Autodesk Fusion 360 part; units mm, degrees
(part 2 of 18)
  line L906 (81.5823, -43.3625) -> (81.9887, -43.0894)
  line L907 (120.3611, -22.6739) -> (127.5638, -15.4712)
  line L908 (99.6621, -41.0408) -> (99.2557, -41.3139)
  line L909 (101.3111, -22.6739) -> (109.1488, -14.8362)
  line L910 (99.2557, -41.3139) -> (98.9843, -41.7214)
  line L911 (62.5323, -60.1036) -> (62.5323, -43.3625)
  line L912 (137.0841, -23.6313) -> (137.3555, -24.0392)
  line L913 (44.2552, -61.2644) -> (44.16, -60.7842)
  line L914 (137.3569, -22.2627) -> (137.0849, -22.6702)
  line L915 (137.3558, -60.3767) -> (137.0844, -60.7842)
  line L916 (81.9887, -43.0894) -> (82.26, -42.6819)
  line L917 (81.9887, -41.3139) -> (81.5823, -41.0408)
  line L918 (117.9391, -23.1507) -> (118.0341, -23.6313)
  line L919 (118.0349, -22.6702) -> (117.9391, -23.1507)
  line L920 (63.3053, -23.1536) -> (63.211, -22.6739)
  line L921 (138.7251, -21.9878) -> (138.2443, -21.8935)
  line L922 (61.562, -43.3625) -> (61.562, -60.1036)
  line L923 (60.8842, -42.6819) -> (61.1556, -43.0894)
  line L924 (42.9971, -81.5853) -> (43.478, -81.4897)
  line L925 (137.0844, -42.6819) -> (137.3558, -43.0894)
  line L926 (61.1556, -60.3767) -> (60.8842, -60.7842)
  line L927 (117.9391, -61.2644) -> (118.0344, -61.7447)
  line L928 (118.0344, -61.7447) -> (118.3057, -62.1522)
  line L929 (118.3052, -79.4399) -> (118.0338, -79.8483)
  line L930 (43.4822, -60.1036) -> (43.4822, -43.3625)
  line L931 (71.8355, -12.6772) -> (62.5249, -21.9878)
  line L932 (98.9843, -61.7447) -> (99.2557, -62.1522)
  line L933 (98.9843, -60.7842) -> (98.8891, -61.2644)
  line L934 (99.2557, -60.3767) -> (98.9843, -60.7842)
  line L935 (99.6621, -43.3625) -> (99.6621, -60.1036)
  line L936 (99.6621, -60.1036) -> (99.2557, -60.3767)
  line L937 (118.7121, -62.4253) -> (118.7121, -79.1663)
  line L938 (99.2555, -24.0392) -> (99.6621, -24.3125)
  line L939 (118.7121, -79.1663) -> (118.3052, -79.4399)
  line L940 (62.9386, -62.1522) -> (63.21, -61.7447)
  line L941 (119.6824, -62.4253) -> (120.0888, -62.1522)
  line L942 (43.8886, -60.3767) -> (43.4822, -60.1036)
  line L943 (42.5119, -79.1663) -> (42.105, -79.4399)
  line L944 (136.9891, -42.2017) -> (137.0844, -42.6819)
  line L945 (98.8891, -61.2644) -> (98.9843, -61.7447)
  line L946 (119.6824, -41.0408) -> (119.6824, -24.3125)
  line L947 (119.6824, -79.1663) -> (119.6824, -62.4253)
  line L948 (120.0888, -62.1522) -> (120.3601, -61.7447)
  line L949 (62.5323, -24.3125) -> (62.9382, -24.0399)
  line L950 (138.2473, -81.5853) -> (138.7282, -81.4897)
  line L951 (63.21, -42.6819) -> (63.3053, -42.2017)
  line L952 (23.0555, -62.1522) -> (23.4619, -62.4253)
  line L953 (23.0555, -60.3767) -> (22.7842, -60.7842)
  line L954 (42.5138, -21.99) -> (42.1067, -22.2627)
  line L955 (24.4322, -41.0408) -> (24.4322, -24.3125)
  line L956 (178.6173, -0.7849) -> (176.3475, -0.7849)
  line L957 (25.2052, -23.1536) -> (25.1109, -22.6739)
  line L958 (23.4661, -81.4897) -> (23.947, -81.5853)
  line L959 (213.072, -5.8134) -> (212.8706, -6.0548)
  line L960 (24.8386, -41.3139) -> (24.4322, -41.0408)
  line L961 (25.2052, -42.2017) -> (25.1099, -41.7214)
  line L962 (41.8342, -60.7842) -> (41.7389, -61.2644)
  line L963 (200.216, -3.6301) -> (200.443, -3.4264)
  line L964 (194.0618, -4.9249) -> (193.7985, -4.9771)
  line L965 (42.1056, -43.0894) -> (42.5119, -43.3625)
  line L966 (4.897, -81.5853) -> (5.378, -81.4897)
  line L967 (176.8325, -43.3625) -> (177.2389, -43.0894)
  line L968 (195.4081, -3.5504) -> (195.6982, -3.4341)
  line L969 (16.129, -12.8042) -> (16.3147, -12.7672)
  line L970 (4.0055, -43.0894) -> (4.4119, -43.3625)
  line L971 (208.5286, -4.7436) -> (208.3683, -4.4841)
  line L972 (172.9629, -1.8839) -> (172.9618, -2.1747)
  line L973 (3.7341, -42.6819) -> (4.0055, -43.0894)
  line L974 (-0.1723, -11.2229) -> (0.0069, -11.7151)
  line L975 (3.7341, -41.7214) -> (3.6389, -42.2017)
  line L976 (215.4944, -11.621) -> (215.6027, -11.9249)
  line L977 (193.4348, -5.3569) -> (190.7733, -5.3569)
  line L978 (200.4816, 0.4328) -> (194.6816, -5.3671)
  line L979 (5.3763, -21.9884) -> (4.8954, -21.8935)
  line L980 (194.9024, -6.8777) -> (201.168, -0.6121)
  line L981 (4.4119, -41.0408) -> (4.0055, -41.3139)
  line L982 (181.9207, 0.92) -> (181.5565, 1.0954)
  line L983 (23.4619, -60.1036) -> (23.0555, -60.3767)
  line L984 (24.428, -81.4897) -> (24.8359, -81.2176)
  line L985 (22.7842, -60.7842) -> (22.6889, -61.2644)
  line L986 (214.101, -6.1558) -> (213.9416, -5.8848)
  line L987 (24.4322, -24.3125) -> (24.8381, -24.0399)
  line L988 (41.8347, -22.6702) -> (41.7389, -23.1507)
  line L989 (216.7062, -11.9249) -> (216.8145, -11.621)
  line L990 (25.1099, -42.6819) -> (25.2052, -42.2017)
  line L991 (203.0295, -6.6507) -> (203.0804, -6.516)
  line L992 (24.4322, -43.3625) -> (24.8386, -43.0894)
  line L993 (25.2052, -80.3294) -> (25.1105, -79.8483)
  line L994 (41.7389, -61.2644) -> (41.8342, -61.7447)
  line L995 (174.114, -1.6018) -> (173.8815, -1.4273)
  line L996 (198.1398, 0.2231) -> (197.8664, 0.2821)
  line L997 (15.9233, -2.4518) -> (15.9041, -2.4514)
  line L998 (173.0884, -1.6216) -> (172.9629, -1.8839)
  line L999 (9.18, -6.8394) -> (8.7726, -7.1123)
  line L1000 (175.2949, -0.9886) -> (175.2326, -1.2915)
  line L1001 (4.0055, -62.1522) -> (4.4119, -62.4253)
  line L1002 (4.0082, -81.2176) -> (4.4161, -81.4897)
  line L1003 (18.072, -9.69) -> (15.9281, -11.8339)
  line L1004 (15.9041, -2.4514) -> (10.8302, -2.4514)
  line L1005 (167.1355, -6.8777) -> (166.9498, -6.9146)
  line L1006 (5.7885, -60.3767) -> (5.3822, -60.1036)
  line L1007 (172.2242, -5.218) -> (172.2313, -5.2888)
  line L1008 (196.8625, -6.7799) -> (196.7084, -6.805)
  line L1009 (8.4049, -8.0011) -> (8.5005, -8.4821)
  line L1010 (195.9027, -3.1978) -> (195.9764, -2.8941)
  line L1011 (4.4119, -62.4253) -> (4.4119, -79.1663)
  line L1012 (3.5508, -9.552) -> (3.0129, -9.4529)
  line L1013 (195.0968, -2.2673) -> (194.8337, -2.436)
  line L1014 (3.7341, -60.7842) -> (3.6389, -61.2644)
  line L1015 (22.7842, -42.6819) -> (23.0555, -43.0894)
  line L1016 (23.0555, -43.0894) -> (23.4619, -43.3625)
  line L1017 (23.4619, -43.3625) -> (23.4619, -60.1036)
  line L1018 (190.7733, -5.3569) -> (190.8695, -5.1322)
  line L1019 (195.0969, -3.521) -> (195.4081, -3.5504)
  line L1020 (41.7389, -42.2017) -> (41.8342, -42.6819)
  line L1021 (207.9228, -5.6157) -> (208.217, -5.5352)
  line L1022 (0.0069, -10.2069) -> (-0.1723, -10.6991)
  line L1023 (180.7794, -1.2929) -> (179.3263, -1.2929)
  line L1024 (190.9024, -3.7901) -> (190.8739, -3.5643)
  line L1025 (15.9424, -2.453) -> (15.9233, -2.4518)
  line L1026 (190.9024, -4.8901) -> (190.9024, -3.7901)
  line L1027 (22.7842, -41.7214) -> (22.6889, -42.2017)
  line L1028 (23.0555, -41.3139) -> (22.7842, -41.7214)
  line L1029 (22.6889, -42.2017) -> (22.7842, -42.6819)
  line L1030 (174.2496, -1.8591) -> (174.114, -1.6018)
  line L1031 (25.1099, -41.7214) -> (24.8386, -41.3139)
  line L1032 (43.4749, -21.9878) -> (42.9941, -21.8935)
  line L1033 (24.4322, -60.1036) -> (24.4322, -43.3625)
  line L1034 (42.1056, -60.3767) -> (41.8342, -60.7842)
  line L1035 (25.1099, -60.7842) -> (24.8386, -60.3767)
  line L1036 (175.2326, -1.2915) -> (175.3144, -1.5898)
  line L1037 (41.8342, -42.6819) -> (42.1056, -43.0894)
  line L1038 (3.6389, -61.2644) -> (3.7341, -61.7447)
  line L1039 (200.6801, 0.5655) -> (200.4816, 0.4328)
  line L1040 (165.1589, -8.4494) -> (165.3162, -8.3442)
  line L1041 (214.3747, -7.2577) -> (214.245, -6.9577)
  line L1042 (3.6389, -80.3294) -> (3.7353, -80.8102)
  line L1043 (5.7891, -79.4399) -> (5.3822, -79.1663)
  line L1044 (15.9425, -3.3693) -> (172.2299, -3.3545)
  line L1045 (198.1837, -6.3551) -> (198.1618, -6.6507)
  line L1046 (172.2242, -3.418) -> (172.2242, -5.218)
  line L1047 (182.2626, -0.59) -> (182.2626, 0.21)
  line L1048 (166.7893, -5.499) -> (164.7723, -7.516)
  line L1049 (5.3822, -43.3625) -> (5.7885, -43.0894)
  line L1050 (6.0599, -60.7842) -> (5.7885, -60.3767)
  line L1051 (16.3147, -12.7672) -> (16.4721, -12.6621)
  line L1052 (198.3525, -0.832) -> (198.7028, -0.925)
  line L1053 (200.1078, -2.4188) -> (199.8039, -2.3916)
  line L1054 (10.1698, -4.0727) -> (10.5742, -3.7888)
  line L1055 (175.7693, -0.6189) -> (175.4878, -0.7469)
  line L1056 (8.5005, -7.5202) -> (8.4049, -8.0011)
  line L1057 (201.688, -1.6181) -> (201.9182, -1.8376)
  line L1058 (23.4619, -24.3125) -> (23.4619, -41.0408)
  line L1059 (5.3822, -41.0408) -> (5.3822, -24.3125)
  line L1060 (22.6889, -80.3294) -> (22.7853, -80.8102)
  line L1061 (23.4619, -41.0408) -> (23.0555, -41.3139)
  line L1062 (197.8664, 0.2821) -> (197.593, 0.2231)
  line L1063 (195.6982, -3.4341) -> (195.9027, -3.1978)
  line L1064 (24.8386, -43.0894) -> (25.1099, -42.6819)
  line L1065 (25.2052, -61.2644) -> (25.1099, -60.7842)
  line L1066 (193.1903, -1.5521) -> (196.8003, -1.5521)
  line L1067 (5.7858, -81.2176) -> (6.0587, -80.8102)
  line L1068 (216.7666, -1.143) -> (216.72, -0.9087)
  line L1069 (179.3263, -1.2929) -> (178.9604, -0.927)
  line L1070 (197.3185, -1.8559) -> (197.6227, -1.8022)
  line L1071 (208.217, -5.5352) -> (208.444, -5.3314)
  line L1072 (216.72, -0.9087) -> (216.5873, -0.7102)
  line L1073 (3.7353, -80.8102) -> (4.0082, -81.2176)
  line L1074 (4.2428, -11.8339) -> (4.4732, -11.3379)
  line L1075 (203.1744, -2.8751) -> (203.3317, -2.9802)
  line L1076 (6.0599, -42.6819) -> (6.1552, -42.2017)
  line L1077 (42.5119, -43.3625) -> (42.5119, -60.1036)
  line L1078 (4.005, -79.4399) -> (3.7336, -79.8483)
  line L1079 (204.1263, -4.4896) -> (203.8403, -4.439)
  line L1080 (18.616, -10.5182) -> (19.9512, -10.5182)
  line L1081 (10.8302, -2.4514) -> (10.5593, -2.0381)
  line L1082 (198.3322, -6.0986) -> (198.1837, -6.3551)
  line L1083 (22.6889, -23.1507) -> (22.7839, -23.6313)
  line L1084 (53.5475, -11.9152) -> (43.4749, -21.9878)
  line L1085 (22.7839, -23.6313) -> (23.0553, -24.0392)
  line L1086 (8.7858, -3.823) -> (9.2008, -4.0913)
  line L1087 (4.0051, -24.039) -> (4.4119, -24.3125)
  line L1088 (24.8386, -62.1522) -> (25.1099, -61.7447)
  line L1089 (10.1419, -9.1646) -> (10.5503, -8.8932)
  line L1090 (24.8386, -60.3767) -> (24.4322, -60.1036)
  line L1091 (23.947, -81.5853) -> (24.428, -81.4897)
  line L1092 (41.8342, -41.7214) -> (41.7389, -42.2017)
  line L1093 (24.4322, -62.4253) -> (24.8386, -62.1522)
  line L1094 (198.0055, -1.3392) -> (198.001, -1.0303)
  line L1095 (5.3822, -60.1036) -> (5.3822, -43.3625)
  line L1096 (6.1552, -61.2644) -> (6.0599, -60.7842)
  line L1097 (5.3822, -79.1663) -> (5.3822, -62.4253)
  line L1098 (180.7882, 0.92) -> (180.5363, 0.6041)
  line L1099 (197.0968, -6.5566) -> (196.8881, -6.7799)
  line L1100 (176.0783, -0.6326) -> (175.7693, -0.6189)
  line L1101 (196.8003, -1.5521) -> (197.023, -1.7661)
  line L1102 (6.0605, -79.8483) -> (5.7891, -79.4399)
  line L1103 (198.3692, -3.9434) -> (198.3322, -4.129)
  line L1104 (200.3673, -2.5791) -> (200.1078, -2.4188)
  line L1105 (3.0129, -9.4529) -> (1.3129, -9.4529)
  line L1106 (16.4721, -12.6621) -> (18.616, -10.5182)
  line L1107 (23.4619, -62.4253) -> (23.4619, -79.1663)
  line L1108 (214.7579, -0.6121) -> (215.5423, -1.3966)
  line L1109 (205.667, -3.1846) -> (205.9467, -3.063)
  line L1110 (42.5119, -60.1036) -> (42.1056, -60.3767)
  line L1111 (4.4119, -43.3625) -> (4.4119, -60.1036)
  line L1112 (189.4281, 0.92) -> (189.1761, 0.6041)
  line L1113 (6.0587, -80.8102) -> (6.1552, -80.3294)
  line L1114 (197.3834, -6.4506) -> (197.0968, -6.5566)
  line L1115 (214.245, -6.9577) -> (213.9877, -6.7562)
  line L1116 (25.1109, -22.6739) -> (35.8696, -11.9152)
  line L1117 (22.7836, -79.8483) -> (22.6889, -80.3294)
  line L1118 (35.8696, -11.9152) -> (53.5475, -11.9152)
  line L1119 (24.8391, -79.4399) -> (24.4322, -79.1663)
  line L1120 (42.9941, -21.8935) -> (42.5138, -21.99)
  line L1121 (10.5742, -3.7888) -> (10.8381, -3.3709)
  line L1122 (25.1099, -61.7447) -> (25.2052, -61.2644)
  line L1123 (25.1105, -79.8483) -> (24.8391, -79.4399)
  line L1124 (42.5119, -41.0408) -> (42.1056, -41.3139)
  line L1125 (5.7885, -43.0894) -> (6.0599, -42.6819)
  line L1126 (200.5548, -3.1425) -> (200.5276, -2.8386)
  line L1127 (195.9764, -2.8941) -> (195.9027, -2.5903)
  line L1128 (199.2151, 0.1448) -> (198.923, 0.3594)
  line L1129 (6.1552, -80.3294) -> (6.0605, -79.8483)
  line L1130 (5.7885, -62.1522) -> (6.0599, -61.7447)
  line L1131 (206.1424, -2.2351) -> (205.9467, -2.0011)
  line L1132 (5.7844, -22.2598) -> (5.3763, -21.9884)
  line L1133 (8.405, -2.9318) -> (8.5061, -3.4155)
  line L1134 (10.8239, -7.516) -> (10.5503, -7.1091)
  line L1135 (201.828, -0.7484) -> (201.637, -1.0027)
  line L1136 (24.8381, -24.0399) -> (25.1094, -23.6331)
  line L1137 (197.023, -1.7661) -> (197.3185, -1.8559)
  line L1138 (194.8337, -2.436) -> (192.3062, -2.4363)
  line L1139 (42.5119, -24.3125) -> (42.5119, -41.0408)
  line L1140 (194.5428, -5.1373) -> (194.3243, -4.9814)
  line L1141 (3.7336, -79.8483) -> (3.6389, -80.3294)
  line L1142 (0.0069, -11.7151) -> (0.3435, -12.1163)
  line L1143 (18.415, -9.5479) -> (18.2294, -9.5848)
  line L1144 (203.7184, -2.0469) -> (202.9101, -1.2386)
  line L1145 (22.7847, -22.6702) -> (22.6889, -23.1507)
  line L1146 (205.9467, -2.0011) -> (205.667, -1.8794)
  line L1147 (23.4619, -79.1663) -> (23.055, -79.4399)
  line L1148 (4.4119, -60.1036) -> (4.0055, -60.3767)
  line L1149 (191.6477, 0.1862) -> (191.4903, 0.081)
  line L1150 (180.4463, 0.21) -> (180.4463, -0.59)
  line L1151 (6.0599, -41.7214) -> (5.7885, -41.3139)
  line L1152 (196.7084, -6.805) -> (196.5703, -6.8777)
  line L1153 (189.2636, -6.5975) -> (189.3011, -6.8777)
  line L1154 (23.4637, -21.99) -> (23.0567, -22.2627)
  line L1155 (23.9441, -21.8935) -> (23.4637, -21.99)
  line L1156 (23.055, -79.4399) -> (22.7836, -79.8483)
  line L1157 (23.0553, -24.0392) -> (23.4619, -24.3125)
  line L1158 (215.4443, 0.4328) -> (215.2457, 0.5655)
  line L1159 (42.1056, -41.3139) -> (41.8342, -41.7214)
  line L1160 (198.5618, 0.3884) -> (198.2393, 0.2231)
  line L1161 (202.1153, -0.6121) -> (201.828, -0.7484)
  line L1162 (8.5061, -3.4155) -> (8.7858, -3.823)
  line L1163 (216.4673, -12.1417) -> (216.7062, -11.9249)
  line L1164 (23.0582, -81.2176) -> (23.4661, -81.4897)
  line L1165 (23.0567, -22.2627) -> (22.7847, -22.6702)
  line L1166 (34.9975, -11.4151) -> (24.4248, -21.9878)
  line L1167 (22.7853, -80.8102) -> (23.0582, -81.2176)
  line L1168 (9.6871, -4.179) -> (10.1698, -4.0727)
  line L1169 (41.834, -23.6313) -> (42.1053, -24.0392)
  line L1170 (199.3507, -0.1912) -> (199.2151, 0.1448)
  line L1171 (175.4878, -0.7469) -> (175.2949, -0.9886)
  line L1172 (196.8881, -6.7799) -> (196.8625, -6.7799)
  line L1173 (1.3129, -9.4529) -> (0.7971, -9.5438)
  line L1174 (199.3163, -2.7304) -> (199.2357, -3.0246)
  line L1175 (24.4248, -21.9878) -> (23.9441, -21.8935)
  line L1176 (23.7467, -11.4151) -> (34.9975, -11.4151)
  line L1177 (23.5871, -11.4421) -> (23.6681, -11.4353)
  line L1178 (182.1727, 0.6041) -> (181.9207, 0.92)
  line L1179 (197.9434, -6.6507) -> (197.6871, -6.4844)
  line L1180 (41.7389, -23.1507) -> (41.834, -23.6313)
  line L1181 (6.0599, -61.7447) -> (6.1552, -61.2644)
  line L1182 (215.2457, 0.5655) -> (215.0114, 0.6121)
  line L1183 (198.4743, -3.786) -> (198.3692, -3.9434)
  line L1184 (3.1779, -12.6621) -> (3.3353, -12.7672)
  line L1185 (23.6681, -11.4353) -> (23.7467, -11.4151)
  line L1186 (20.3591, -11.4421) -> (23.5871, -11.4421)
  line L1187 (8.1491, -23.5999) -> (8.3065, -23.4947)
  line L1188 (25.1094, -23.6331) -> (25.2052, -23.1536)
  line L1189 (203.7228, -4.386) -> (203.5951, -4.3679)
  line L1190 (208.1088, -4.3238) -> (207.8049, -4.2966)
  line L1191 (193.5774, -5.1294) -> (193.4348, -5.3569)
  line L1192 (9.18, -9.1629) -> (9.6608, -9.2593)
  line L1193 (9.6608, -6.743) -> (9.18, -6.8394)
  line L1194 (7.7625, -22.6665) -> (6.0579, -22.6665)
  line L1195 (199.9607, -4.0327) -> (199.7531, -4.2406)
  line L1196 (10.5593, -2.0381) -> (10.1501, -1.7611)
  line L1197 (166.9467, -5.3938) -> (166.7893, -5.499)
  line L1198 (7.9634, -23.6368) -> (8.1491, -23.5999)
  line L1199 (8.3065, -23.4947) -> (20.3591, -11.4421)
  line L1200 (22.7842, -61.7447) -> (23.0555, -62.1522)
  line L1201 (207.1669, -6.1706) -> (207.3526, -6.1337)
  line L1202 (200.7795, -4.1206) -> (200.5297, -3.9662)
  line L1203 (42.1053, -24.0392) -> (42.5119, -24.3125)
  line L1204 (198.923, 0.3594) -> (198.5618, 0.3884)
  line L1205 (6.1552, -42.2017) -> (6.0599, -41.7214)
  line L1206 (4.4119, -79.1663) -> (4.005, -79.4399)
  line L1207 (174.3183, -1.9279) -> (174.2496, -1.8591)
  line L1208 (207.2367, -4.9296) -> (206.966, -5.2003)
  line L1209 (3.7337, -23.6309) -> (4.0051, -24.039)
  line L1210 (5.7867, -24.0413) -> (6.0579, -23.6368)
  line L1211 (5.3822, -24.3125) -> (5.7867, -24.0413)
  line L1212 (22.6889, -61.2644) -> (22.7842, -61.7447)
  line L1213 (4.0179, -9.8365) -> (3.5508, -9.552)
  line L1214 (25.1088, -80.8102) -> (25.2052, -80.3294)
  line L1215 (4.0055, -60.3767) -> (3.7341, -60.7842)
  line L1216 (24.4322, -79.1663) -> (24.4322, -62.4253)
  line L1217 (24.8359, -81.2176) -> (25.1088, -80.8102)
  line L1218 (42.1067, -22.2627) -> (41.8347, -22.6702)
  line L1219 (207.5211, -4.4084) -> (207.3173, -4.6354)
  line L1220 (203.5951, -4.3679) -> (200.9382, -4.3679)
  line L1221 (189.0861, -0.59) -> (189.1736, -0.9789)
  line L1222 (5.3822, -62.4253) -> (5.7885, -62.1522)
  line L1223 (203.0804, -6.516) -> (203.1011, -6.3734)
  line L1224 (191.8334, 0.2231) -> (191.6477, 0.1862)
  line L1225 (212.803, -6.3619) -> (212.5142, -6.6507)
  line L1226 (213.8751, -8.0076) -> (214.1642, -7.8552)
  line L1227 (4.4732, -11.3379) -> (4.5116, -10.7923)
  line L1228 (3.7341, -61.7447) -> (4.0055, -62.1522)
  line L1229 (173.0851, -2.4381) -> (15.9424, -2.453)
  line L1230 (5.378, -81.4897) -> (5.7858, -81.2176)
  line L1231 (192.3062, -2.4363) -> (193.1903, -1.5521)
  line L1232 (19.879, -10.5602) -> (19.8151, -10.6139)
  line L1233 (206.1424, -2.8289) -> (206.2125, -2.532)
  line L1234 (0.3435, -9.8057) -> (0.0069, -10.2069)
  line L1235 (6.0579, -23.6368) -> (7.9634, -23.6368)
  line L1236 (4.4161, -81.4897) -> (4.897, -81.5853)
  line L1237 (203.5174, -3.0171) -> (205.0973, -3.0171)
  line L1238 (5.7885, -41.3139) -> (5.3822, -41.0408)
  line L1239 (189.4193, -1.2929) -> (181.9295, -1.2929)
  line L1240 (213.362, -5.6919) -> (213.072, -5.8134)
  line L1241 (4.3529, -10.2689) -> (4.0179, -9.8365)
  line L1242 (1.8785, -81.4188) -> (1.397, -81.323)
  line L1243 (0.5074, -81.6915) -> (0.2346, -82.0997)
  line L1244 (0.9155, -83.7435) -> (1.397, -83.8393)
  line L1245 (2.5594, -82.0997) -> (2.2866, -81.6915)
  line L1246 (1.397, -81.323) -> (0.9155, -81.4188)
  line L1247 (2.2866, -83.4708) -> (2.5594, -83.0626)
  line L1248 (1.397, -83.8393) -> (1.8785, -83.7435)
  line L1249 (2.6551, -82.5812) -> (2.5594, -82.0997)
  line L1250 (0.1389, -82.5812) -> (0.2346, -83.0626)
  line L1251 (0.2346, -82.0997) -> (0.1389, -82.5812)
  line L1252 (0.2346, -83.0626) -> (0.5074, -83.4708)
  line L1253 (1.8785, -83.7435) -> (2.2866, -83.4708)
  line L1254 (2.2866, -81.6915) -> (1.8785, -81.4188)
  line L1255 (2.5594, -83.0626) -> (2.6551, -82.5812)
  line L1256 (0.5074, -83.4708) -> (0.9155, -83.7435)
  line L1257 (0.9155, -81.4188) -> (0.5074, -81.6915)
  line L1258 (1.8785, -64.6808) -> (2.2866, -64.4081)
  line L1259 (0.5074, -64.4081) -> (0.9155, -64.6808)
  line L1260 (2.2866, -62.6288) -> (1.8785, -62.3561)
  line L1261 (0.5074, -62.6288) -> (0.2346, -63.037)
  line L1262 (2.6551, -63.5184) -> (2.5594, -63.037)
  line L1263 (2.5594, -63.9999) -> (2.6551, -63.5184)
  line L1264 (0.2346, -63.037) -> (0.1389, -63.5184)
  line L1265 (0.2346, -63.9999) -> (0.5074, -64.4081)
  line L1266 (0.9155, -64.6808) -> (1.397, -64.7766)
  line L1267 (2.5594, -63.037) -> (2.2866, -62.6288)
  line L1268 (0.1389, -63.5184) -> (0.2346, -63.9999)
  line L1269 (0.9155, -62.3561) -> (0.5074, -62.6288)
  line L1270 (1.8785, -62.3561) -> (1.397, -62.2603)
  line L1271 (1.397, -64.7766) -> (1.8785, -64.6808)
  line L1272 (2.2866, -64.4081) -> (2.5594, -63.9999)
  line L1273 (1.397, -62.2603) -> (0.9155, -62.3561)
  line L1274 (0.5074, -26.2953) -> (0.9155, -26.568)
  line L1275 (0.9155, -26.568) -> (1.397, -26.6638)
  line L1276 (2.2866, -24.516) -> (1.8785, -24.2433)
  line L1277 (2.5594, -24.9242) -> (2.2866, -24.516)
  line L1278 (0.2346, -24.9242) -> (0.1389, -25.4057)
  line L1279 (1.397, -24.1475) -> (0.9155, -24.2433)
  line L1280 (0.9155, -24.2433) -> (0.5074, -24.516)
  line L1281 (1.397, -26.6638) -> (1.8785, -26.568)
  line L1282 (2.2866, -26.2953) -> (2.5594, -25.8871)
  line L1283 (2.6551, -25.4057) -> (2.5594, -24.9242)
  line L1284 (1.8785, -26.568) -> (2.2866, -26.2953)
  line L1285 (0.5074, -24.516) -> (0.2346, -24.9242)
  line L1286 (1.8785, -24.2433) -> (1.397, -24.1475)
  line L1287 (2.5594, -25.8871) -> (2.6551, -25.4057)
  line L1288 (0.2346, -25.8871) -> (0.5074, -26.2953)
  line L1289 (0.1389, -25.4057) -> (0.2346, -25.8871)
  line L1290 (2.5594, -44.9372) -> (2.6551, -44.4557)
  line L1291 (0.5074, -43.566) -> (0.2346, -43.9742)
  line L1292 (2.2866, -43.566) -> (1.8785, -43.2933)
  line L1293 (1.8785, -45.6181) -> (2.2866, -45.3453)
  line L1294 (0.2346, -43.9742) -> (0.1389, -44.4557)
  line L1295 (0.9155, -45.6181) -> (1.397, -45.7138)
  line L1296 (2.2866, -45.3453) -> (2.5594, -44.9372)
  line L1297 (1.397, -43.1975) -> (0.9155, -43.2933)
  line L1298 (0.5074, -45.3453) -> (0.9155, -45.6181)
  line L1299 (0.2346, -44.9372) -> (0.5074, -45.3453)
  line L1300 (1.397, -45.7138) -> (1.8785, -45.6181)
  line L1301 (0.1389, -44.4557) -> (0.2346, -44.9372)
  line L1302 (2.6551, -44.4557) -> (2.5594, -43.9742)
  line L1303 (2.5594, -43.9742) -> (2.2866, -43.566)
  line L1304 (1.8785, -43.2933) -> (1.397, -43.1975)
  line L1305 (0.9155, -43.2933) -> (0.5074, -43.566)
  line L1306 (9.1816, -4.2988) -> (8.7734, -4.5715)
  line L1307 (10.9212, -5.4611) -> (10.8254, -4.9797)
  line L1308 (8.4049, -5.4611) -> (8.5007, -5.9426)
  line L1309 (10.8254, -4.9797) -> (10.5527, -4.5715)
  line L1310 (10.8254, -5.9426) -> (10.9212, -5.4611)
  line L1311 (8.7734, -6.3508) -> (9.1816, -6.6235)
  line L1312 (8.7734, -4.5715) -> (8.5007, -4.9797)
  line L1313 (10.5527, -4.5715) -> (10.1445, -4.2988)
  line L1314 (10.5527, -6.3508) -> (10.8254, -5.9426)
  line L1315 (10.1445, -6.6235) -> (10.5527, -6.3508)
  line L1316 (8.5007, -5.9426) -> (8.7734, -6.3508)
  line L1317 (10.1445, -4.2988) -> (9.6631, -4.203)
  line L1318 (9.6631, -4.203) -> (9.1816, -4.2988)
  line L1319 (9.6631, -6.7193) -> (10.1445, -6.6235)
  line L1320 (8.5007, -4.9797) -> (8.4049, -5.4611)
  line L1321 (9.1816, -6.6235) -> (9.6631, -6.7193)
  line L1322 (17.6863, -18.6659) -> (17.5889, -19.4056)
  line L1323 (17.5889, -19.4056) -> (17.6863, -20.1454)
  line L1324 (19.7073, -22.1664) -> (20.447, -22.2638)
  line L1325 (22.4681, -21.4267) -> (22.9223, -20.8347)
  line L1326 (23.2078, -20.1454) -> (23.3052, -19.4056)
  line L1327 (21.8761, -16.9304) -> (21.1868, -16.6449)
  line L1328 (23.2078, -18.6659) -> (22.9223, -17.9766)
  line L1329 (18.426, -17.3846) -> (17.9718, -17.9766)
  line L1330 (22.4681, -17.3846) -> (21.8761, -16.9304)
  line L1331 (19.018, -21.8809) -> (19.7073, -22.1664)
  line L1332 (21.1868, -22.1664) -> (21.8761, -21.8809)
  line L1333 (22.9223, -20.8347) -> (23.2078, -20.1454)
  line L1334 (18.426, -21.4267) -> (19.018, -21.8809)
  line L1335 (22.9223, -17.9766) -> (22.4681, -17.3846)
  line L1336 (17.6863, -20.1454) -> (17.9718, -20.8347)
  line L1337 (21.8761, -21.8809) -> (22.4681, -21.4267)
  line L1338 (21.1868, -16.6449) -> (20.447, -16.5475)
  line L1339 (19.018, -16.9304) -> (18.426, -17.3846)
  line L1340 (17.9718, -17.9766) -> (17.6863, -18.6659)
  line L1341 (20.447, -22.2638) -> (21.1868, -22.1664)
  line L1342 (20.447, -16.5475) -> (19.7073, -16.6449)
  line L1343 (19.7073, -16.6449) -> (19.018, -16.9304)
  line L1344 (23.3052, -19.4056) -> (23.2078, -18.6659)
  line L1345 (17.9718, -20.8347) -> (18.426, -21.4267)
  line L1346 (21.8761, -74.1059) -> (21.1868, -73.8204)
  line L1347 (22.9223, -75.1521) -> (22.4681, -74.5601)
  line L1348 (17.6863, -77.3209) -> (17.9718, -78.0102)
  line L1349 (17.9718, -78.0102) -> (18.426, -78.6022)
  line L1350 (20.447, -79.4393) -> (21.1868, -79.3419)
  line L1351 (19.018, -74.1059) -> (18.426, -74.5601)
  line L1352 (19.018, -79.0564) -> (19.7073, -79.3419)
  line L1353 (21.1868, -79.3419) -> (21.8761, -79.0564)
  line L1354 (19.7073, -73.8204) -> (19.018, -74.1059)
  line L1355 (21.8761, -79.0564) -> (22.4681, -78.6022)
  line L1356 (18.426, -74.5601) -> (17.9718, -75.1521)
  line L1357 (17.6863, -75.8414) -> (17.5889, -76.5812)
  line L1358 (17.5889, -76.5812) -> (17.6863, -77.3209)
  line L1359 (23.3052, -76.5812) -> (23.2078, -75.8414)
  line L1360 (17.9718, -75.1521) -> (17.6863, -75.8414)
  line L1361 (19.7073, -79.3419) -> (20.447, -79.4393)
  line L1362 (22.9223, -78.0102) -> (23.2078, -77.3209)
  line L1363 (22.4681, -78.6022) -> (22.9223, -78.0102)
  line L1364 (20.447, -73.723) -> (19.7073, -73.8204)
  line L1365 (21.1868, -73.8204) -> (20.447, -73.723)
  line L1366 (22.4681, -74.5601) -> (21.8761, -74.1059)
  line L1367 (23.2078, -75.8414) -> (22.9223, -75.1521)
  line L1368 (23.2078, -77.3209) -> (23.3052, -76.5812)
  line L1369 (18.426, -78.6022) -> (19.018, -79.0564)
  line L1370 (23.2078, -37.7159) -> (22.9223, -37.0266)
  line L1371 (19.7073, -35.6949) -> (19.018, -35.9805)
  line L1372 (17.6863, -37.7159) -> (17.5889, -38.4557)
  line L1373 (19.018, -35.9805) -> (18.426, -36.4347)
  line L1374 (18.426, -40.4767) -> (19.018, -40.9309)
  line L1375 (23.2078, -39.1954) -> (23.3052, -38.4557)
  line L1376 (17.9718, -37.0266) -> (17.6863, -37.7159)
  line L1377 (22.4681, -40.4767) -> (22.9223, -39.8847)
  line L1378 (23.3052, -38.4557) -> (23.2078, -37.7159)
  line L1379 (17.5889, -38.4557) -> (17.6863, -39.1954)
  line L1380 (20.447, -35.5975) -> (19.7073, -35.6949)
  line L1381 (18.426, -36.4347) -> (17.9718, -37.0266)
  line L1382 (19.018, -40.9309) -> (19.7073, -41.2164)
  line L1383 (20.447, -41.3138) -> (21.1868, -41.2164)
  line L1384 (22.4681, -36.4347) -> (21.8761, -35.9805)
  line L1385 (22.9223, -37.0266) -> (22.4681, -36.4347)
  line L1386 (21.1868, -35.6949) -> (20.447, -35.5975)
  line L1387 (17.6863, -39.1954) -> (17.9718, -39.8847)
  line L1388 (21.8761, -40.9309) -> (22.4681, -40.4767)
  line L1389 (21.8761, -35.9805) -> (21.1868, -35.6949)
  line L1390 (17.9718, -39.8847) -> (18.426, -40.4767)
  line L1391 (19.7073, -41.2164) -> (20.447, -41.3138)
  line L1392 (21.1868, -41.2164) -> (21.8761, -40.9309)
  line L1393 (22.9223, -39.8847) -> (23.2078, -39.1954)
  line L1394 (22.4681, -59.5394) -> (22.9223, -58.9475)
  line L1395 (17.5889, -57.5184) -> (17.6863, -58.2582)
  line L1396 (20.447, -60.3766) -> (21.1868, -60.2792)
  line L1397 (23.2078, -58.2582) -> (23.3052, -57.5184)
  line L1398 (23.2078, -56.7787) -> (22.9223, -56.0893)
  line L1399 (21.1868, -60.2792) -> (21.8761, -59.9936)
  line L1400 (19.7073, -54.7577) -> (19.018, -55.0432)
  line L1401 (19.7073, -60.2792) -> (20.447, -60.3766)
  line L1402 (21.1868, -54.7577) -> (20.447, -54.6603)
  line L1403 (17.6863, -58.2582) -> (17.9718, -58.9475)
  line L1404 (18.426, -55.4974) -> (17.9718, -56.0893)
  line L1405 (17.6863, -56.7787) -> (17.5889, -57.5184)
  line L1406 (19.018, -59.9936) -> (19.7073, -60.2792)
  line L1407 (17.9718, -56.0893) -> (17.6863, -56.7787)
  line L1408 (21.8761, -55.0432) -> (21.1868, -54.7577)
  line L1409 (22.9223, -58.9475) -> (23.2078, -58.2582)
  line L1410 (18.426, -59.5394) -> (19.018, -59.9936)
  line L1411 (22.4681, -55.4974) -> (21.8761, -55.0432)
  line L1412 (17.9718, -58.9475) -> (18.426, -59.5394)
  line L1413 (22.9223, -56.0893) -> (22.4681, -55.4974)
  line L1414 (19.018, -55.0432) -> (18.426, -55.4974)
  line L1415 (20.447, -54.6603) -> (19.7073, -54.7577)
  line L1416 (21.8761, -59.9936) -> (22.4681, -59.5394)
  line L1417 (23.3052, -57.5184) -> (23.2078, -56.7787)
  line L1418 (19.9656, -81.4188) -> (19.5574, -81.6915)
  line L1419 (19.2847, -83.0626) -> (19.5574, -83.4708)
  line L1420 (21.3367, -83.4708) -> (21.6094, -83.0626)
  line L1421 (20.9285, -81.4188) -> (20.447, -81.323)
  line L1422 (20.9285, -83.7435) -> (21.3367, -83.4708)
  line L1423 (21.6094, -82.0997) -> (21.3367, -81.6915)
  line L1424 (19.2847, -82.0997) -> (19.1889, -82.5812)
  line L1425 (21.6094, -83.0626) -> (21.7052, -82.5812)
  line L1426 (20.447, -81.323) -> (19.9656, -81.4188)
  line L1427 (19.5574, -83.4708) -> (19.9656, -83.7435)
  line L1428 (19.9656, -83.7435) -> (20.447, -83.8393)
  line L1429 (21.7052, -82.5812) -> (21.6094, -82.0997)
  line L1430 (21.3367, -81.6915) -> (20.9285, -81.4188)
  line L1431 (20.447, -83.8393) -> (20.9285, -83.7435)
  line L1432 (19.5574, -81.6915) -> (19.2847, -82.0997)
  line L1433 (19.1889, -82.5812) -> (19.2847, -83.0626)
  line L1434 (19.5574, -64.4081) -> (19.9656, -64.6808)
  line L1435 (19.2847, -63.037) -> (19.1889, -63.5184)
  line L1436 (20.9285, -64.6808) -> (21.3367, -64.4081)
  line L1437 (20.9285, -62.3561) -> (20.447, -62.2603)
  line L1438 (21.7052, -63.5184) -> (21.6094, -63.037)
  line L1439 (19.5574, -62.6288) -> (19.2847, -63.037)
  line L1440 (20.447, -64.7766) -> (20.9285, -64.6808)
  line L1441 (21.3367, -62.6288) -> (20.9285, -62.3561)
  line L1442 (21.3367, -64.4081) -> (21.6094, -63.9999)
  line L1443 (21.6094, -63.9999) -> (21.7052, -63.5184)
  line L1444 (19.2847, -63.9999) -> (19.5574, -64.4081)
  line L1445 (19.9656, -64.6808) -> (20.447, -64.7766)
  line L1446 (19.1889, -63.5184) -> (19.2847, -63.9999)
  line L1447 (19.9656, -62.3561) -> (19.5574, -62.6288)
  line L1448 (21.6094, -63.037) -> (21.3367, -62.6288)
  line L1449 (20.447, -62.2603) -> (19.9656, -62.3561)
  line L1450 (21.6094, -25.8871) -> (21.7052, -25.4057)
  line L1451 (19.9656, -26.568) -> (20.447, -26.6638)
  line L1452 (19.9656, -24.2433) -> (19.5574, -24.516)
  line L1453 (19.2847, -25.8871) -> (19.5574, -26.2953)
  line L1454 (20.9285, -24.2433) -> (20.447, -24.1475)
  line L1455 (19.2847, -24.9242) -> (19.1889, -25.4057)
  line L1456 (19.1889, -25.4057) -> (19.2847, -25.8871)
  line L1457 (20.447, -24.1475) -> (19.9656, -24.2433)
  line L1458 (19.5574, -26.2953) -> (19.9656, -26.568)
  line L1459 (21.6094, -24.9242) -> (21.3367, -24.516)
  line L1460 (20.9285, -26.568) -> (21.3367, -26.2953)
  line L1461 (20.447, -26.6638) -> (20.9285, -26.568)
  line L1462 (21.7052, -25.4057) -> (21.6094, -24.9242)
  line L1463 (21.3367, -24.516) -> (20.9285, -24.2433)
  line L1464 (19.5574, -24.516) -> (19.2847, -24.9242)
  line L1465 (21.3367, -26.2953) -> (21.6094, -25.8871)
  line L1466 (19.2847, -43.9742) -> (19.1889, -44.4557)
  line L1467 (19.2847, -44.9372) -> (19.5574, -45.3453)
  line L1468 (21.3367, -45.3453) -> (21.6094, -44.9372)
  line L1469 (19.9656, -43.2933) -> (19.5574, -43.566)
  line L1470 (20.9285, -43.2933) -> (20.447, -43.1975)
  line L1471 (20.447, -43.1975) -> (19.9656, -43.2933)
  line L1472 (20.9285, -45.6181) -> (21.3367, -45.3453)
  line L1473 (21.7052, -44.4557) -> (21.6094, -43.9742)
  line L1474 (20.447, -45.7138) -> (20.9285, -45.6181)
  line L1475 (21.6094, -44.9372) -> (21.7052, -44.4557)
  line L1476 (19.5574, -45.3453) -> (19.9656, -45.6181)
  line L1477 (21.6094, -43.9742) -> (21.3367, -43.566)
  line L1478 (21.3367, -43.566) -> (20.9285, -43.2933)
  line L1479 (19.9656, -45.6181) -> (20.447, -45.7138)
  line L1480 (19.5574, -43.566) -> (19.2847, -43.9742)
  line L1481 (19.1889, -44.4557) -> (19.2847, -44.9372)
  line L1482 (42.3552, -19.4056) -> (42.2578, -18.6659)
  line L1483 (42.2578, -18.6659) -> (41.9723, -17.9766)
  line L1484 (39.4971, -16.5475) -> (38.7573, -16.6449)
  line L1485 (38.7573, -22.1664) -> (39.4971, -22.2638)
  line L1486 (37.4761, -17.3846) -> (37.0219, -17.9766)
  line L1487 (38.068, -16.9304) -> (37.4761, -17.3846)
  line L1488 (36.7363, -20.1454) -> (37.0219, -20.8347)
  line L1489 (36.6389, -19.4056) -> (36.7363, -20.1454)
  line L1490 (41.9723, -17.9766) -> (41.5181, -17.3846)
  line L1491 (38.7573, -16.6449) -> (38.068, -16.9304)
  line L1492 (40.9262, -21.8809) -> (41.5181, -21.4267)
  line L1493 (38.068, -21.8809) -> (38.7573, -22.1664)
  line L1494 (40.2368, -16.6449) -> (39.4971, -16.5475)
  line L1495 (37.0219, -17.9766) -> (36.7363, -18.6659)
  line L1496 (41.5181, -21.4267) -> (41.9723, -20.8347)
  line L1497 (37.0219, -20.8347) -> (37.4761, -21.4267)
  line L1498 (37.4761, -21.4267) -> (38.068, -21.8809)
  line L1499 (40.2368, -22.1664) -> (40.9262, -21.8809)
  line L1500 (41.9723, -20.8347) -> (42.2578, -20.1454)
  line L1501 (36.7363, -18.6659) -> (36.6389, -19.4056)
  line L1502 (42.2578, -20.1454) -> (42.3552, -19.4056)
  line L1503 (40.9262, -16.9304) -> (40.2368, -16.6449)
  line L1504 (39.4971, -22.2638) -> (40.2368, -22.1664)
  line L1505 (41.5181, -17.3846) -> (40.9262, -16.9304)
  line L1506 (41.5181, -78.6022) -> (41.9723, -78.0102)
  line L1507 (40.9262, -74.1059) -> (40.2368, -73.8204)
  line L1508 (42.2578, -77.3209) -> (42.3552, -76.5812)
  line L1509 (42.3552, -76.5812) -> (42.2578, -75.8414)
  line L1510 (36.7363, -75.8414) -> (36.6389, -76.5812)
  line L1511 (39.4971, -73.723) -> (38.7573, -73.8204)
  line L1512 (37.0219, -78.0102) -> (37.4761, -78.6022)
  line L1513 (36.7363, -77.3209) -> (37.0219, -78.0102)
  line L1514 (39.4971, -79.4393) -> (40.2368, -79.3419)
  line L1515 (38.7573, -73.8204) -> (38.068, -74.1059)
  line L1516 (41.9723, -78.0102) -> (42.2578, -77.3209)
  line L1517 (38.7573, -79.3419) -> (39.4971, -79.4393)
  line L1518 (36.6389, -76.5812) -> (36.7363, -77.3209)
  line L1519 (40.2368, -73.8204) -> (39.4971, -73.723)
  line L1520 (42.2578, -75.8414) -> (41.9723, -75.1521)
  line L1521 (38.068, -74.1059) -> (37.4761, -74.5601)
  line L1522 (38.068, -79.0564) -> (38.7573, -79.3419)
  line L1523 (37.4761, -78.6022) -> (38.068, -79.0564)
  line L1524 (40.9262, -79.0564) -> (41.5181, -78.6022)
  line L1525 (41.5181, -74.5601) -> (40.9262, -74.1059)
  line L1526 (41.9723, -75.1521) -> (41.5181, -74.5601)
  line L1527 (37.4761, -74.5601) -> (37.0219, -75.1521)
  line L1528 (40.2368, -79.3419) -> (40.9262, -79.0564)
  line L1529 (37.0219, -75.1521) -> (36.7363, -75.8414)
  line L1530 (41.5181, -40.4767) -> (41.9723, -39.8847)
  line L1531 (42.2578, -39.1954) -> (42.3552, -38.4557)
  line L1532 (37.0219, -39.8847) -> (37.4761, -40.4767)
  line L1533 (41.9723, -37.0266) -> (41.5181, -36.4347)
  line L1534 (40.9262, -40.9309) -> (41.5181, -40.4767)
  line L1535 (39.4971, -41.3138) -> (40.2368, -41.2164)
  line L1536 (36.6389, -38.4557) -> (36.7363, -39.1954)
  line L1537 (37.4761, -40.4767) -> (38.068, -40.9309)
  line L1538 (38.7573, -35.6949) -> (38.068, -35.9805)
  line L1539 (37.0219, -37.0266) -> (36.7363, -37.7159)
  line L1540 (36.7363, -39.1954) -> (37.0219, -39.8847)
  line L1541 (40.9262, -35.9805) -> (40.2368, -35.6949)
  line L1542 (39.4971, -35.5975) -> (38.7573, -35.6949)
  line L1543 (41.9723, -39.8847) -> (42.2578, -39.1954)
  line L1544 (41.5181, -36.4347) -> (40.9262, -35.9805)
  line L1545 (42.2578, -37.7159) -> (41.9723, -37.0266)
  line L1546 (38.068, -40.9309) -> (38.7573, -41.2164)
  line L1547 (36.7363, -37.7159) -> (36.6389, -38.4557)
  line L1548 (40.2368, -41.2164) -> (40.9262, -40.9309)
  line L1549 (42.3552, -38.4557) -> (42.2578, -37.7159)
  line L1550 (38.7573, -41.2164) -> (39.4971, -41.3138)
  line L1551 (38.068, -35.9805) -> (37.4761, -36.4347)
  line L1552 (37.4761, -36.4347) -> (37.0219, -37.0266)
  line L1553 (40.2368, -35.6949) -> (39.4971, -35.5975)
  line L1554 (40.2368, -54.7577) -> (39.4971, -54.6603)
  line L1555 (38.7573, -60.2792) -> (39.4971, -60.3766)
  line L1556 (38.7573, -54.7577) -> (38.068, -55.0432)
  line L1557 (36.7363, -56.7787) -> (36.6389, -57.5184)
  line L1558 (39.4971, -54.6603) -> (38.7573, -54.7577)
  line L1559 (41.5181, -59.5394) -> (41.9723, -58.9475)
  line L1560 (41.9723, -56.0893) -> (41.5181, -55.4974)
  line L1561 (40.2368, -60.2792) -> (40.9262, -59.9936)
  line L1562 (40.9262, -55.0432) -> (40.2368, -54.7577)
  line L1563 (38.068, -59.9936) -> (38.7573, -60.2792)
  line L1564 (41.9723, -58.9475) -> (42.2578, -58.2582)
  line L1565 (36.7363, -58.2582) -> (37.0219, -58.9475)
  line L1566 (42.2578, -58.2582) -> (42.3552, -57.5184)
  line L1567 (38.068, -55.0432) -> (37.4761, -55.4974)
  line L1568 (40.9262, -59.9936) -> (41.5181, -59.5394)
  line L1569 (42.2578, -56.7787) -> (41.9723, -56.0893)
  line L1570 (42.3552, -57.5184) -> (42.2578, -56.7787)
  line L1571 (37.4761, -55.4974) -> (37.0219, -56.0893)
  line L1572 (37.0219, -56.0893) -> (36.7363, -56.7787)
  line L1573 (39.4971, -60.3766) -> (40.2368, -60.2792)
  line L1574 (37.0219, -58.9475) -> (37.4761, -59.5394)
  line L1575 (41.5181, -55.4974) -> (40.9262, -55.0432)
  line L1576 (37.4761, -59.5394) -> (38.068, -59.9936)
  line L1577 (36.6389, -57.5184) -> (36.7363, -58.2582)
  line L1578 (38.6074, -83.4708) -> (39.0156, -83.7435)
  line L1579 (39.9785, -81.4188) -> (39.4971, -81.323)
  line L1580 (40.6595, -83.0626) -> (40.7552, -82.5812)
  line L1581 (39.4971, -81.323) -> (39.0156, -81.4188)
  line L1582 (38.2389, -82.5812) -> (38.3347, -83.0626)
  line L1583 (38.3347, -82.0997) -> (38.2389, -82.5812)
  line L1584 (40.3867, -83.4708) -> (40.6595, -83.0626)
  line L1585 (40.7552, -82.5812) -> (40.6595, -82.0997)
  line L1586 (38.6074, -81.6915) -> (38.3347, -82.0997)
  line L1587 (39.4971, -83.8393) -> (39.9785, -83.7435)
  line L1588 (38.3347, -83.0626) -> (38.6074, -83.4708)
  line L1589 (40.6595, -82.0997) -> (40.3867, -81.6915)
  line L1590 (39.9785, -83.7435) -> (40.3867, -83.4708)
  line L1591 (40.3867, -81.6915) -> (39.9785, -81.4188)
  line L1592 (39.0156, -81.4188) -> (38.6074, -81.6915)
  line L1593 (39.0156, -83.7435) -> (39.4971, -83.8393)
  line L1594 (38.2389, -63.5184) -> (38.3347, -63.9999)
  line L1595 (39.4971, -62.2603) -> (39.0156, -62.3561)
  line L1596 (40.3867, -64.4081) -> (40.6595, -63.9999)
  line L1597 (39.0156, -64.6808) -> (39.4971, -64.7766)
  line L1598 (39.4971, -64.7766) -> (39.9785, -64.6808)
  line L1599 (38.6074, -62.6288) -> (38.3347, -63.037)
  line L1600 (40.6595, -63.037) -> (40.3867, -62.6288)
  line L1601 (40.7552, -63.5184) -> (40.6595, -63.037)
  line L1602 (40.3867, -62.6288) -> (39.9785, -62.3561)
  line L1603 (39.0156, -62.3561) -> (38.6074, -62.6288)
  line L1604 (38.6074, -64.4081) -> (39.0156, -64.6808)
  line L1605 (38.3347, -63.9999) -> (38.6074, -64.4081)
  line L1606 (38.3347, -63.037) -> (38.2389, -63.5184)
  line L1607 (40.6595, -63.9999) -> (40.7552, -63.5184)
  line L1608 (39.9785, -64.6808) -> (40.3867, -64.4081)
  line L1609 (39.9785, -62.3561) -> (39.4971, -62.2603)
  line L1610 (40.3867, -24.516) -> (39.9785, -24.2433)
  line L1611 (38.6074, -24.516) -> (38.3347, -24.9242)
  line L1612 (39.9785, -24.2433) -> (39.4971, -24.1475)
  line L1613 (38.3347, -25.8871) -> (38.6074, -26.2953)
  line L1614 (39.9785, -26.568) -> (40.3867, -26.2953)
  line L1615 (39.0156, -24.2433) -> (38.6074, -24.516)
  line L1616 (40.6595, -24.9242) -> (40.3867, -24.516)
  line L1617 (39.4971, -24.1475) -> (39.0156, -24.2433)
  line L1618 (39.0156, -26.568) -> (39.4971, -26.6638)
  line L1619 (38.2389, -25.4057) -> (38.3347, -25.8871)
  line L1620 (40.3867, -26.2953) -> (40.6595, -25.8871)
  line L1621 (40.7552, -25.4057) -> (40.6595, -24.9242)
  line L1622 (40.6595, -25.8871) -> (40.7552, -25.4057)
  line L1623 (39.4971, -26.6638) -> (39.9785, -26.568)
  line L1624 (38.6074, -26.2953) -> (39.0156, -26.568)
  line L1625 (38.3347, -24.9242) -> (38.2389, -25.4057)
  line L1626 (40.3867, -43.566) -> (39.9785, -43.2933)
  line L1627 (40.7552, -44.4557) -> (40.6595, -43.9742)
  line L1628 (38.6074, -45.3453) -> (39.0156, -45.6181)
  line L1629 (38.3347, -43.9742) -> (38.2389, -44.4557)
  line L1630 (39.4971, -45.7138) -> (39.9785, -45.6181)
  line L1631 (39.0156, -45.6181) -> (39.4971, -45.7138)
  line L1632 (39.4971, -43.1975) -> (39.0156, -43.2933)
  line L1633 (40.6595, -44.9372) -> (40.7552, -44.4557)
  line L1634 (40.6595, -43.9742) -> (40.3867, -43.566)
  line L1635 (39.0156, -43.2933) -> (38.6074, -43.566)
  line L1636 (38.2389, -44.4557) -> (38.3347, -44.9372)
  line L1637 (39.9785, -43.2933) -> (39.4971, -43.1975)
  line L1638 (38.6074, -43.566) -> (38.3347, -43.9742)
  line L1639 (40.3867, -45.3453) -> (40.6595, -44.9372)
  line L1640 (38.3347, -44.9372) -> (38.6074, -45.3453)
  line L1641 (39.9785, -45.6181) -> (40.3867, -45.3453)
  line L1642 (56.0719, -20.8347) -> (56.5261, -21.4267)
  line L1643 (61.3079, -20.1454) -> (61.4053, -19.4056)
  line L1644 (58.5471, -22.2638) -> (59.2869, -22.1664)
  line L1645 (55.689, -19.4056) -> (55.7864, -20.1454)
  line L1646 (59.2869, -22.1664) -> (59.9762, -21.8809)
  line L1647 (61.3079, -18.6659) -> (61.0223, -17.9766)
  line L1648 (56.5261, -21.4267) -> (57.118, -21.8809)
  line L1649 (61.4053, -19.4056) -> (61.3079, -18.6659)
  line L1650 (55.7864, -20.1454) -> (56.0719, -20.8347)
  line L1651 (57.118, -21.8809) -> (57.8074, -22.1664)
  line L1652 (58.5471, -16.5475) -> (57.8074, -16.6449)
  line L1653 (61.0223, -20.8347) -> (61.3079, -20.1454)
  line L1654 (59.9762, -21.8809) -> (60.5681, -21.4267)
  line L1655 (60.5681, -17.3846) -> (59.9762, -16.9304)
  line L1656 (59.2869, -16.6449) -> (58.5471, -16.5475)
  line L1657 (57.8074, -16.6449) -> (57.118, -16.9304)
  line L1658 (56.0719, -17.9766) -> (55.7864, -18.6659)
  line L1659 (57.8074, -22.1664) -> (58.5471, -22.2638)
  line L1660 (55.7864, -18.6659) -> (55.689, -19.4056)
  line L1661 (60.5681, -21.4267) -> (61.0223, -20.8347)
  line L1662 (56.5261, -17.3846) -> (56.0719, -17.9766)
  line L1663 (61.0223, -17.9766) -> (60.5681, -17.3846)
  line L1664 (57.118, -16.9304) -> (56.5261, -17.3846)
  line L1665 (59.9762, -16.9304) -> (59.2869, -16.6449)
  line L1666 (56.0719, -78.0102) -> (56.5261, -78.6022)
  line L1667 (61.3079, -75.8414) -> (61.0223, -75.1521)
  line L1668 (56.5261, -78.6022) -> (57.118, -79.0564)
  line L1669 (58.5471, -73.723) -> (57.8074, -73.8204)
  line L1670 (57.118, -79.0564) -> (57.8074, -79.3419)
  line L1671 (57.8074, -79.3419) -> (58.5471, -79.4393)
  line L1672 (60.5681, -74.5601) -> (59.9762, -74.1059)
  line L1673 (58.5471, -79.4393) -> (59.2869, -79.3419)
  line L1674 (56.5261, -74.5601) -> (56.0719, -75.1521)
  line L1675 (60.5681, -78.6022) -> (61.0223, -78.0102)
  line L1676 (55.7864, -75.8414) -> (55.689, -76.5812)
  line L1677 (57.8074, -73.8204) -> (57.118, -74.1059)
  line L1678 (61.0223, -75.1521) -> (60.5681, -74.5601)
  line L1679 (59.2869, -79.3419) -> (59.9762, -79.0564)
  line L1680 (59.9762, -79.0564) -> (60.5681, -78.6022)
  line L1681 (61.0223, -78.0102) -> (61.3079, -77.3209)
  line L1682 (61.4053, -76.5812) -> (61.3079, -75.8414)
  line L1683 (59.9762, -74.1059) -> (59.2869, -73.8204)
  line L1684 (57.118, -74.1059) -> (56.5261, -74.5601)
  line L1685 (61.3079, -77.3209) -> (61.4053, -76.5812)
  line L1686 (55.689, -76.5812) -> (55.7864, -77.3209)
  line L1687 (59.2869, -73.8204) -> (58.5471, -73.723)
  line L1688 (56.0719, -75.1521) -> (55.7864, -75.8414)
  line L1689 (55.7864, -77.3209) -> (56.0719, -78.0102)
  line L1690 (55.689, -38.4557) -> (55.7864, -39.1954)
  line L1691 (57.8074, -41.2164) -> (58.5471, -41.3138)
  line L1692 (56.5261, -40.4767) -> (57.118, -40.9309)
  line L1693 (58.5471, -41.3138) -> (59.2869, -41.2164)
  line L1694 (56.0719, -39.8847) -> (56.5261, -40.4767)
  line L1695 (57.118, -40.9309) -> (57.8074, -41.2164)
  line L1696 (55.7864, -39.1954) -> (56.0719, -39.8847)
  line L1697 (59.9762, -35.9805) -> (59.2869, -35.6949)
  line L1698 (59.2869, -41.2164) -> (59.9762, -40.9309)
  line L1699 (58.5471, -35.5975) -> (57.8074, -35.6949)
  line L1700 (57.118, -35.9805) -> (56.5261, -36.4347)
  line L1701 (60.5681, -36.4347) -> (59.9762, -35.9805)
  line L1702 (56.0719, -37.0266) -> (55.7864, -37.7159)
  line L1703 (61.0223, -37.0266) -> (60.5681, -36.4347)
  line L1704 (61.3079, -37.7159) -> (61.0223, -37.0266)
  line L1705 (61.3079, -39.1954) -> (61.4053, -38.4557)
  line L1706 (61.0223, -39.8847) -> (61.3079, -39.1954)
  line L1707 (56.5261, -36.4347) -> (56.0719, -37.0266)
  line L1708 (59.9762, -40.9309) -> (60.5681, -40.4767)
  line L1709 (59.2869, -35.6949) -> (58.5471, -35.5975)
  line L1710 (57.8074, -35.6949) -> (57.118, -35.9805)
  line L1711 (61.4053, -38.4557) -> (61.3079, -37.7159)
  line L1712 (60.5681, -40.4767) -> (61.0223, -39.8847)
  line L1713 (55.7864, -37.7159) -> (55.689, -38.4557)
  line L1714 (55.7864, -58.2582) -> (56.0719, -58.9475)
  line L1715 (56.0719, -56.0893) -> (55.7864, -56.7787)
  line L1716 (58.5471, -54.6603) -> (57.8074, -54.7577)
  line L1717 (55.689, -57.5184) -> (55.7864, -58.2582)
  line L1718 (55.7864, -56.7787) -> (55.689, -57.5184)
  line L1719 (61.4053, -57.5184) -> (61.3079, -56.7787)
  line L1720 (57.118, -55.0432) -> (56.5261, -55.4974)
  line L1721 (56.0719, -58.9475) -> (56.5261, -59.5394)
  line L1722 (56.5261, -55.4974) -> (56.0719, -56.0893)
  line L1723 (57.8074, -54.7577) -> (57.118, -55.0432)
  line L1724 (59.2869, -54.7577) -> (58.5471, -54.6603)
  line L1725 (61.3079, -58.2582) -> (61.4053, -57.5184)
  line L1726 (58.5471, -60.3766) -> (59.2869, -60.2792)
  line L1727 (61.3079, -56.7787) -> (61.0223, -56.0893)
  line L1728 (59.9762, -59.9936) -> (60.5681, -59.5394)
  line L1729 (61.0223, -56.0893) -> (60.5681, -55.4974)
  line L1730 (61.0223, -58.9475) -> (61.3079, -58.2582)
  line L1731 (59.2869, -60.2792) -> (59.9762, -59.9936)
  line L1732 (59.9762, -55.0432) -> (59.2869, -54.7577)
  line L1733 (56.5261, -59.5394) -> (57.118, -59.9936)
  line L1734 (57.8074, -60.2792) -> (58.5471, -60.3766)
  line L1735 (60.5681, -55.4974) -> (59.9762, -55.0432)
  line L1736 (60.5681, -59.5394) -> (61.0223, -58.9475)
  line L1737 (57.118, -59.9936) -> (57.8074, -60.2792)
  line L1738 (59.4368, -81.6915) -> (59.0286, -81.4188)
  line L1739 (57.3847, -83.0626) -> (57.6575, -83.4708)
  line L1740 (58.0656, -83.7435) -> (58.5471, -83.8393)
  line L1741 (57.3847, -82.0997) -> (57.289, -82.5812)
  line L1742 (59.7095, -82.0997) -> (59.4368, -81.6915)
  line L1743 (59.4368, -83.4708) -> (59.7095, -83.0626)
  line L1744 (57.289, -82.5812) -> (57.3847, -83.0626)
  line L1745 (58.0656, -81.4188) -> (57.6575, -81.6915)
  line L1746 (58.5471, -83.8393) -> (59.0286, -83.7435)
  line L1747 (58.5471, -81.323) -> (58.0656, -81.4188)
  line L1748 (59.7095, -83.0626) -> (59.8053, -82.5812)
  line L1749 (57.6575, -81.6915) -> (57.3847, -82.0997)
  line L1750 (59.0286, -83.7435) -> (59.4368, -83.4708)
  line L1751 (59.0286, -81.4188) -> (58.5471, -81.323)
  line L1752 (57.6575, -83.4708) -> (58.0656, -83.7435)
  line L1753 (59.8053, -82.5812) -> (59.7095, -82.0997)
  line L1754 (57.289, -63.5184) -> (57.3847, -63.9999)
  line L1755 (57.6575, -64.4081) -> (58.0656, -64.6808)
  line L1756 (59.7095, -63.9999) -> (59.8053, -63.5184)
  line L1757 (59.7095, -63.037) -> (59.4368, -62.6288)
  line L1758 (58.5471, -64.7766) -> (59.0286, -64.6808)
  line L1759 (58.0656, -64.6808) -> (58.5471, -64.7766)
  line L1760 (59.4368, -64.4081) -> (59.7095, -63.9999)
  line L1761 (57.6575, -62.6288) -> (57.3847, -63.037)
  line L1762 (58.5471, -62.2603) -> (58.0656, -62.3561)
  line L1763 (59.4368, -62.6288) -> (59.0286, -62.3561)
  line L1764 (59.0286, -64.6808) -> (59.4368, -64.4081)
  line L1765 (59.0286, -62.3561) -> (58.5471, -62.2603)
  line L1766 (57.3847, -63.037) -> (57.289, -63.5184)
  line L1767 (57.3847, -63.9999) -> (57.6575, -64.4081)
  line L1768 (58.0656, -62.3561) -> (57.6575, -62.6288)
  line L1769 (59.8053, -63.5184) -> (59.7095, -63.037)
  line L1770 (59.7095, -25.8871) -> (59.8053, -25.4057)
  line L1771 (59.4368, -24.516) -> (59.0286, -24.2433)
  line L1772 (59.4368, -26.2953) -> (59.7095, -25.8871)
  line L1773 (57.6575, -26.2953) -> (58.0656, -26.568)
  line L1774 (59.8053, -25.4057) -> (59.7095, -24.9242)
  line L1775 (58.0656, -24.2433) -> (57.6575, -24.516)
  line L1776 (59.0286, -24.2433) -> (58.5471, -24.1475)
  line L1777 (58.0656, -26.568) -> (58.5471, -26.6638)
  line L1778 (58.5471, -26.6638) -> (59.0286, -26.568)
  line L1779 (57.3847, -24.9242) -> (57.289, -25.4057)
  line L1780 (57.289, -25.4057) -> (57.3847, -25.8871)
  line L1781 (59.7095, -24.9242) -> (59.4368, -24.516)
  line L1782 (57.6575, -24.516) -> (57.3847, -24.9242)
  line L1783 (58.5471, -24.1475) -> (58.0656, -24.2433)
  line L1784 (57.3847, -25.8871) -> (57.6575, -26.2953)
  line L1785 (59.0286, -26.568) -> (59.4368, -26.2953)
  line L1786 (57.289, -44.4557) -> (57.3847, -44.9372)
  line L1787 (57.3847, -43.9742) -> (57.289, -44.4557)
  line L1788 (59.8053, -44.4557) -> (59.7095, -43.9742)
  line L1789 (57.3847, -44.9372) -> (57.6575, -45.3453)
  line L1790 (59.7095, -43.9742) -> (59.4368, -43.566)
  line L1791 (59.0286, -43.2933) -> (58.5471, -43.1975)
  line L1792 (58.5471, -45.7138) -> (59.0286, -45.6181)
  line L1793 (59.4368, -43.566) -> (59.0286, -43.2933)
  line L1794 (57.6575, -45.3453) -> (58.0656, -45.6181)
  line L1795 (58.0656, -43.2933) -> (57.6575, -43.566)
  line L1796 (59.0286, -45.6181) -> (59.4368, -45.3453)
  line L1797 (59.4368, -45.3453) -> (59.7095, -44.9372)
  line L1798 (58.0656, -45.6181) -> (58.5471, -45.7138)
  line L1799 (59.7095, -44.9372) -> (59.8053, -44.4557)
  line L1800 (57.6575, -43.566) -> (57.3847, -43.9742)
  line L1801 (58.5471, -43.1975) -> (58.0656, -43.2933)
  line L1802 (80.0724, -20.8347) -> (80.3579, -20.1454)
  line L1803 (80.4553, -19.4056) -> (80.3579, -18.6659)
  line L1804 (80.0724, -17.9766) -> (79.6182, -17.3846)
  line L1805 (74.8364, -18.6659) -> (74.739, -19.4056)
  line L1806 (78.3369, -22.1664) -> (79.0262, -21.8809)
  line L1807 (77.5972, -16.5475) -> (76.8574, -16.6449)
  line L1808 (79.0262, -21.8809) -> (79.6182, -21.4267)
  line L1809 (79.6182, -21.4267) -> (80.0724, -20.8347)
  line L1810 (75.5761, -17.3846) -> (75.1219, -17.9766)